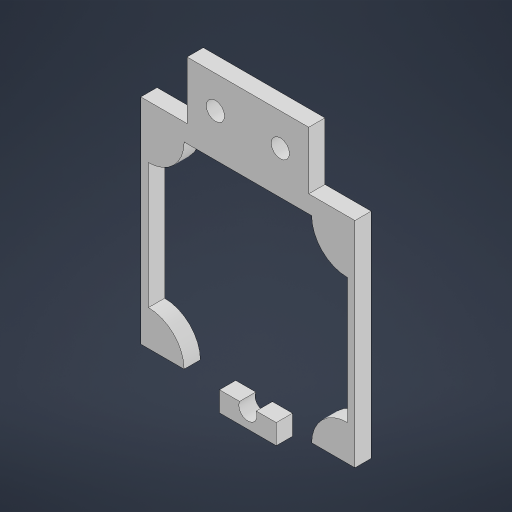
# Autodesk Inventor part: Clamp connector 2
Saved by Autodesk Inventor 2024 (Build 280153000, 153)
## iProperties
Created: 2024-02-01
Part Number: Clamp connector 2
Material: Generic
Document SubType Name: Modeling
Designer: chenq
Density: 1 g/cm^3
Appearance: Default
Author: chenq
Autodesk Inventor part; units mm, degrees
ref_plane "YZ Plane" through (0, 0, 0) normal (1, 0, 0) x (0, 1, 0)
ref_plane "XZ Plane" through (0, 0, 0) normal (0, 1, 0) x (-1, 0, 0)
ref_plane "XY Plane" through (0, 0, 0) normal (0, 0, 1) x (1, 0, 0)
sketch "Sketch1" plane through (0, 0, 0) normal (0, 0, 1) x (1, 0, 0)
  line L0 (0, 0) -> (47.625, 0)
  line L1 (47.625, 0) -> (47.625, 22.5806)
  line L2 (47.625, 22.5806) -> (0, 22.5806)
  line L3 (0, 22.5806) -> (0, 0)
  line L4 (23.8125, 22.5806) -> (23.8125, 9.8806)
  line L5 (23.8125, 9.8806) -> (36.5125, 9.8806)
  line L6 (23.8125, 9.8806) -> (11.1125, 9.8806)
  circle A0 centre (11.1125, 9.8806) radius 3.5687
  circle A1 centre (36.5125, 9.8806) radius 3.5687
  dimension "d1" = 47.625
  dimension "d3" = 12.7
  dimension "d4" = 12.7
  dimension "d5" = 12.7
  dimension "d6" = 7.1374
  dimension "d7" = 7.1374
  dimension "d10" = 22.5806
  constraints: 14 end point, 2 centre point, 2 coincident, 2 horizontal, 2 parallel, 2 perpendicular, 1 midpoint, 1 vertical
  measures "d1" distance of L1.end L2.end
  measures "d3" distance of L4.start L4.end
  measures "d4" distance of L4.end L5.end
  measures "d5" distance of L4.end L6.end
  measures "d6" diameter of A0
  measures "d7" diameter of A1
  measures "d10" distance of L0.end L1.end
extrude "Extrusion1" add sketch "Sketch1" along normal blind 6.35
sketch "Sketch3" plane through (0, 0, 6.35) normal (0, 0, 1) x (1, 0, 0)
  line L0 (0, 0) -> (47.625, 0) projected
  line L1 (23.8125, 0) -> (65.7225, 0)
  line L2 (23.8125, 0) -> (23.8125, -41.91)
  circle A0 centre (23.8125, -41.91) radius 33.02
  line L3 (65.7225, 0) -> (-18.0975, 0)
  line L4 (-18.0975, 0) -> (-18.0975, -83.82)
  line L5 (-18.0975, -83.82) -> (65.7225, -83.82)
  line L6 (65.7225, -83.82) -> (65.7225, 0)
  circle A1 centre (11.1125, 9.8806) radius 3.5687 projected
  line L7 (23.8125, 9.8806) -> (23.8125, -85.3694)
  line L8 (23.8125, 9.8806) -> (119.0625, 9.8806) construction
  line L9 (11.1125, 9.8806) -> (23.8125, 9.8806)
  circle A2 centre (23.8125, -85.3694) radius 3.5687
  line L10 (12.7, -91.7194) -> (34.925, -91.7194)
  line L11 (34.925, -91.7194) -> (34.925, -79.0194)
  line L12 (34.925, -79.0194) -> (12.7, -79.0194)
  line L13 (12.7, -79.0194) -> (12.7, -91.7194)
  line L14 (12.7, -91.7194) -> (34.925, -79.0194) construction
  line L15 (34.925, -91.7194) -> (12.7, -79.0194) construction
  point P0 (12.7, -83.82)
  point P1 (34.925, -83.82)
  dimension "d11" = 41.91
  dimension "d12" = 41.91
  dimension "d13" = 66.04
  dimension "d14" = 83.82
  dimension "d15" = 83.82
  dimension "d18" = 95.25
  dimension "d19" = 90
  dimension "d20" = 7.1374
  dimension "d22" = 22.225
  dimension "d23" = 12.7
  constraints: 30 end point, 4 horizontal, 4 parallel, 3 midpoint, 3 perpendicular, 2 centre point, 2 coincident, 2 vertical, 1 collinear
  measures "d11" distance of L1.start L1.end
  measures "d12" distance of L1.start L2.end
  measures "d13" diameter of A0
  measures "d14" distance of L5.end L4.end
  measures "d15" distance of L4.end L3.end
  measures "d18" distance of L7.start L7.end
  measures "d19" angle of L7 L8
  measures "d20" diameter of A2
  measures "d22" distance of L11.end L12.end
  measures "d23" distance of L10.end L11.end
extrude "Extrusion2" add sketch "Sketch3" against normal blind 6.35 contours L0 L2 A0 L7 L12 L13 L5 L4 L3 | L0 L1 L6 L5 L11 L12 L7 A0 L2 | L13 L12 L7 A2 L5 | L5 A2 L11 L10 L13 | L12 L11 L5 A2 L7
sketch "Sketch4" plane through (0, 0, 0) normal (0, 0, -1) x (-1, 0, 0)
  line L0 (-47.625, 22.5806) -> (0, 22.5806) projected
  line L1 (-23.8125, 22.5806) -> (-23.8125, 0)
  line L2 (-23.8125, 0) -> (-23.8125, -6.8072)
  line L3 (-23.8125, -6.8072) -> (1.143, -6.8072)
  line L4 (-23.8125, -6.8072) -> (-48.7807, -6.8072)
  line L5 (-48.7807, -6.8072) -> (-62.7507, -6.8072)
  line L6 (1.143, -6.8072) -> (15.113, -6.8072)
  line L7 (-62.7507, -6.8072) -> (-62.7507, -20.7772)
  arc A0 (-62.7507, -20.7772) -> (-48.7807, -6.8072) centre (-62.7507, -6.8072) ccw
  line L8 (-62.7507, -20.7772) -> (-62.7507, -45.3517)
  line L9 (-62.7507, -45.3517) -> (8.128, -45.3517)
  line L10 (15.113, -6.8072) -> (15.113, -20.7772)
  arc A1 (1.143, -6.8072) -> (15.113, -20.7772) centre (15.113, -6.8072) ccw
  line L11 (15.113, -20.7772) -> (15.113, -45.3644)
  line L12 (-23.8125, -83.8962) -> (1.143, -83.8962)
  line L13 (-23.8125, -83.8962) -> (-48.7807, -83.8962)
  arc A2 (-48.7807, -83.8962) -> (-62.7507, -69.9262) centre (-62.7507, -83.8962) ccw
  line L14 (-62.7507, -69.9262) -> (-62.7507, -45.3517)
  arc A3 (15.113, -69.9262) -> (1.143, -83.8962) centre (15.113, -83.8962) ccw
  line L15 (15.113, -69.9262) -> (15.113, -45.339)
  point P0 (0, 0)
  dimension "d26" = 6.8072
  dimension "d27" = 24.9555
  dimension "d28" = 24.9682
  dimension "d29" = 13.97
  dimension "d30" = 13.97
  dimension "d31" = 13.97
  dimension "d32" = 13.97
  dimension "d33" = 24.5745
  dimension "d34" = 13.97
  dimension "d35" = 13.97
  dimension "d36" = 24.5872
  constraints: 30 end point, 8 point on circle, 8 symmetric about line, 5 horizontal, 5 vertical, 4 centre point, 1 midpoint, 1 point on line, 2 other
  measures "d26" distance of L1.end L2.end
  measures "d27" distance of L2.end L3.end
  measures "d28" distance of L2.end L4.end
  measures "d29" distance of L4.end L5.end
  measures "d30" distance of L3.end L6.end
  measures "d31" distance of L5.end L7.end
  measures "d32" radius of A0
  measures "d33" distance of L7.end L8.end
  measures "d34" distance of L6.end L10.end
  measures "d35" radius of A1
  measures "d36" distance of L10.end L11.end
extrude "Extrusion3" cut sketch "Sketch4" against normal blind 6.35 contours L3 A1 L11 L15 A3 L12 L13 A2 L14 L8 A0 L4
body "Solid1"
